Autodesk Fusion 360 part; units mm, degrees
note: some values were not read from the file. Chosen so that the rebuilt part matches the saved one: which bodies a step acts on.
(part 3 of 3)
  arc A214 (-6.6815, -293.4215) -> (-18.1828, -272.523) centre (-11.8765, -282.6665) cw
  arc A215 (-11.8752, -478.4075) -> (-10.2989, -476.8852) centre (3.5069, -492.7565) cw
  arc A216 (-159.2076, -214.1306) -> (-165.4906, -200.711) centre (-150.5091, -201.8774) cw
  arc A217 (-116.8581, -195.2756) -> (-109.0263, -217.8093) centre (-113.5449, -206.7519) cw
  arc A218 (-10.2989, -476.8852) -> (14.3752, -490.0489) centre (-0.5458, -488.3104) cw
  arc A219 (-16.473, -529.8025) -> (-27.9743, -508.904) centre (-21.668, -519.0474) cw
  arc A220 (47.4338, -419.9097) -> (41.1509, -406.49) centre (56.1324, -407.6565) cw
  arc A221 (-141.5323, -182.1119) -> (-116.8581, -195.2756) centre (-131.7791, -193.5371) cw
  arc A222 (-90.0824, -111.7167) -> (-76.5895, -97.9367) centre (-75.1054, -112.8859) cw
  arc A223 (-83.7995, -125.1364) -> (-90.0824, -111.7167) centre (-75.1009, -112.8832) cw
  line L0 (-266.5509, -596.9) -> (-266.5509, 0)
  arc A224 (266.8491, -596.9) -> (-266.5509, -596.9) centre (0.1491, -596.9) cw
  line L1 (266.8491, 0) -> (266.8491, -596.9)
  line L2 (241.4491, 0) -> (266.8491, 0)
  line L3 (-241.1509, 0) -> (-241.1509, -411.8539)
  arc A225 (-241.1509, -596.9) -> (241.4491, -596.9) centre (0.1491, -596.9) ccw
  line L4 (-241.1509, -439.1647) -> (-241.1509, -596.9)
  line L5 (241.4491, -596.9) -> (241.4491, 0)
  line L6 (-215.7509, -25.4) -> (-215.7509, -420.1147)
  arc A226 (-215.7509, -596.9) -> (216.0491, -596.9) centre (0.1491, -596.9) ccw
  line L7 (216.0491, -596.9) -> (216.0491, -25.4)
  line L8 (-215.7509, -439.1647) -> (-215.7509, -596.9)
  line L9 (-190.3509, -50.8) -> (-190.3509, -420.1147)
  line L10 (190.6491, -596.9) -> (190.6491, -50.8)
  line L11 (-190.3509, -439.1647) -> (-190.3509, -596.9)
  arc A227 (-190.3509, -596.9) -> (190.6491, -596.9) centre (0.1491, -596.9) ccw
  line L12 (216.0491, -25.4) -> (-215.7509, -25.4)
  line L13 (190.6491, -50.8) -> (-190.3509, -50.8)
  circle A228 centre (-203.0509, -429.6397) radius 6.35
  line L14 (-260.2009, -411.8539) -> (-241.1509, -411.8539)
  line L15 (-241.1509, -411.8539) -> (-241.1509, -428.0522)
  line L16 (-241.1509, -428.0522) -> (-260.2009, -428.0522)
  line L17 (-260.2009, -428.0522) -> (-260.2009, -411.8539)
  arc A229 (-152.1305, -436.5446) -> (-151.004, -435.1368) centre (-151.705, -435.7305) ccw
  line L18 (-261.7725, -439.1647) -> (-186.7302, -439.1647)
  arc A230 (-184.4429, -438.341) -> (-152.1305, -436.5446) centre (-167.2009, -456.9736) cw
  line L19 (-260.2009, -420.1147) -> (-261.7725, -420.1147)
  line L20 (-181.8374, -420.1147) -> (-241.1509, -420.1147)
  arc A231 (-151.004, -435.1368) -> (-181.8374, -420.1147) centre (-180.7971, -457.1339) ccw
  arc A232 (-261.7725, -420.1147) -> (-261.7725, -439.1647) centre (-236.358, -429.6397) ccw
  arc A233 (-186.7302, -439.1647) -> (-184.4429, -438.341) centre (-186.7379, -435.5556) ccw
  line L21 (222.3991, -25.4) -> (235.0991, -25.4)
  line L22 (235.0991, -25.4) -> (235.0991, -101.6)
  line L23 (235.0991, -101.6) -> (222.3991, -101.6)
  line L24 (222.3991, -101.6) -> (222.3991, -25.4)
  line L25 (222.3991, -63.5) -> (235.0991, -63.5)
  line L26 (216.0491, -25.4) -> (216.0491, -63.5)
  line L27 (216.0491, -63.5) -> (222.3991, -63.5)
  line L28 (222.3991, -63.5) -> (222.3991, -25.4)
  line L29 (222.3991, -25.4) -> (216.0491, -25.4)
  line L30 (235.0991, -101.6) -> (241.4491, -101.6)
  line L31 (235.0991, -63.5) -> (235.0991, -101.6)
  line L32 (241.4491, -63.5) -> (235.0991, -63.5)
  line L33 (241.4491, -101.6) -> (241.4491, -63.5)
  line L34 (222.3991, -518.7254) -> (235.0991, -518.7254)
  line L35 (235.0991, -594.9254) -> (222.3991, -594.9254)
  line L36 (222.3991, -594.9254) -> (222.3991, -518.7254)
  line L37 (235.0991, -518.7254) -> (235.0991, -594.9254)
  line L38 (222.3991, -556.8254) -> (235.0991, -556.8254)
  line L39 (216.0491, -518.7254) -> (216.0491, -556.8254)
  line L40 (222.3991, -556.8254) -> (222.3991, -518.7254)
  line L41 (222.3991, -518.7254) -> (216.0491, -518.7254)
  line L42 (216.0491, -556.8254) -> (222.3991, -556.8254)
  line L43 (241.4491, -556.8254) -> (235.0991, -556.8254)
  line L44 (235.0991, -556.8254) -> (235.0991, -594.9254)
  line L45 (235.0991, -594.9254) -> (241.4491, -594.9254)
  line L46 (241.4491, -594.9254) -> (241.4491, -556.8254)
  line L47 (6.4991, -50.8) -> (6.4991, -237.1607)
  line L48 (6.4991, -242.0445) -> (6.4991, -277.5095)
  line L49 (6.4991, -282.0442) -> (6.4991, -295.7652)
  line L50 (6.4991, -300.6585) -> (6.4991, -475.0428)
  line L51 (6.4991, -480.8522) -> (6.4991, -496.4423)
  line L52 (6.4991, -512.5757) -> (6.4991, -522.9778)
  line L53 (6.4991, -528.6458) -> (6.4991, -787.2941)
  line L54 (-6.2009, -50.8) -> (-6.2009, -244.5718)
  line L55 (-6.2009, -249.5407) -> (-6.2009, -272.1568)
  line L56 (-6.2009, -278.266) -> (-6.2009, -287.0667)
  line L57 (-6.2009, -294.4545) -> (-6.2009, -474.3935)
  line L58 (-6.2009, -479.7502) -> (-6.2009, -514.0409)
  line L59 (-6.2009, -518.147) -> (-6.2009, -532.4242)
  line L60 (-6.2009, -537.2039) -> (-6.2009, -787.2941)
  line L61 (-59.1175, -50.8) -> (-59.1175, -89.7741)
  line L62 (-59.1175, -94.6578) -> (-59.1175, -130.1228)
  line L63 (-59.1175, -134.6575) -> (-59.1175, -148.3785)
  line L64 (-59.1175, -153.2719) -> (-59.1175, -327.6562)
  line L65 (-59.1175, -333.4655) -> (-59.1175, -349.0556)
  line L66 (-59.1175, -365.1891) -> (-59.1175, -375.5911)
  line L67 (-59.1175, -381.2592) -> (-59.1175, -777.9462)
  line L68 (-71.8175, -50.8) -> (-71.8175, -97.1851)
  line L69 (-71.8175, -102.1541) -> (-71.8175, -124.5061)
  line L70 (-71.8175, -130.8793) -> (-71.8175, -139.68)
  line L71 (-71.8175, -147.0678) -> (-71.8175, -327.0069)
  line L72 (-71.8175, -332.3636) -> (-71.8175, -366.6542)
  line L73 (-71.8175, -370.7604) -> (-71.8175, -385.0376)
  line L74 (-71.8175, -389.8173) -> (-71.8175, -773.2832)
  line L75 (72.1158, -50.8) -> (72.1158, -384.5474)
  line L76 (72.1158, -389.4311) -> (72.1158, -424.8962)
  line L77 (72.1158, -429.4308) -> (72.1158, -443.1518)
  line L78 (72.1158, -448.0452) -> (72.1158, -622.4295)
  line L79 (72.1158, -628.2388) -> (72.1158, -643.8289)
  line L80 (72.1158, -659.9624) -> (72.1158, -670.3644)
  line L81 (72.1158, -676.0325) -> (72.1158, -773.2832)
  line L82 (59.4158, -50.8) -> (59.4158, -391.9584)
  line L83 (59.4158, -396.9274) -> (59.4158, -419.5435)
  line L84 (59.4158, -425.6526) -> (59.4158, -434.4533)
  line L85 (59.4158, -441.8411) -> (59.4158, -621.7802)
  line L86 (59.4158, -627.1369) -> (59.4158, -661.4275)
  line L87 (59.4158, -665.5337) -> (59.4158, -679.8109)
  line L88 (59.4158, -684.5906) -> (59.4158, -777.9462)
  line L89 (137.7325, -50.8) -> (137.7325, -531.934)
  line L90 (137.7325, -536.8178) -> (137.7325, -572.2828)
  line L91 (137.7325, -576.8175) -> (137.7325, -590.5385)
  line L92 (137.7325, -595.4318) -> (137.7325, -728.6614)
  line L93 (125.0325, -50.8) -> (125.0325, -539.3451)
  line L94 (125.0325, -544.314) -> (125.0325, -566.6661)
  line L95 (125.0325, -573.0393) -> (125.0325, -581.84)
  line L96 (125.0325, -589.2278) -> (125.0325, -740.7555)
  line L97 (-124.7342, -50.8) -> (-124.7342, -180.2695)
  line L98 (-124.7342, -186.0789) -> (-124.7342, -201.669)
  line L99 (-124.7342, -217.8024) -> (-124.7342, -228.2045)
  line L100 (-124.7342, -233.8725) -> (-124.7342, -740.7555)
  line L101 (-137.4342, -50.8) -> (-137.4342, -179.6202)
  line L102 (-137.4342, -184.9769) -> (-137.4342, -219.2676)
  line L103 (-137.4342, -223.3737) -> (-137.4342, -237.6509)
  line L104 (-137.4342, -242.4306) -> (-137.4342, -728.6614)
  line L105 (284.6029, 0) -> (-289.1743, 0)
extrude "Extrude5" add sketch "DJ - Baxley - Dog Door (1) (curves -6.35 mm off its plane)" against normal blind 6.35 separate body contours A8 A16 A62 A142 A214 | A8 A54 A142 L55 | A8 A32 A43 A48 A50 A54 A62 A63 A76 A99 A102 A112 A113 A115 A176 A177 A188 A191 A193 A196 A211 L55 | A8 A16 A32 A146 | A8 A16 A32 A62 | A10 A35 A45 A58 A65 A68 A69 A74 A77 A87 A88 A96 A106 A107 A121 A152 A155 A199 A200 A212 A215 A218 | A16 A32 A43 A62 A207 | A17 A35 A45 A121 A210 | A9 A39 A47 A109 A111 A118 A119 A120 A123 A126 A136 A137 A139 A140 A143 A169 A185 A189 A192 A194 A222 A223 | A12 A34 A41 A64 A66 A67 A70 A80 A81 A90 A93 A95 A103 A117 A144 A150 A203 A208 A209 A213 A220 L83 | A10 A17 A35 A153 | A10 A17 A87 A121 A219 | A14 A38 A46 A110 A114 A116 A122 A124 A125 A127 A130 A131 A132 A133 A135 A174 A201 A205 A206 A216 A217 A221 | A22 A39 A47 A109 A171 | A10 A17 A35 A121 | A13 A36 A44 A51 A59 A60 A73 A75 A84 A86 A97 A98 A101 A105 A128 A147 A148 A151 A158 A161 A164 A170 | A11 A19 A33 A162 | A20 A34 A41 A70 A154 | A21 A38 A46 A124 A198 | A9 A22 A39 A195 | A23 A37 A40 A55 A183 | A19 A33 A42 A53 A163 | A11 A19 A49 A53 A168 | A12 A20 A70 A91 A202 | A9 A22 A109 A123 A197 | A15 A23 A37 A182 | A13 A18 A36 A160 | A11 A33 A42 A49 A52 A53 A71 A78 A82 A83 A94 A100 A104 A138 A141 A145 A149 A156 A157 A159 A165 A167 | A18 A36 A44 A73 A172 | A12 A20 A34 A204 | A12 A81 A91 L83 | A9 A22 A39 A109 | A15 A37 A40 A55 A56 A57 A61 A72 A79 A85 A89 A92 A108 A129 A134 A173 A175 A179 A180 A181 A187 A190 | A15 A23 A55 A61 A184 | A13 A18 A73 A128 A166 | A11 A19 A33 A53 | A14 A21 A38 A186 | A15 A23 A37 A55 | A12 A20 A34 A70 | A14 A21 A38 A124 | A14 A21 A124 A135 A178 | A13 A18 A36 A73 makes body 4 at (76.4475, -6.35, 427.4285) makes body 5 at (1.0394, -6.35, 516.4228) makes body 6 at (10.8309, -6.35, 280.0418) makes body 7 at (142.0642, -6.35, 574.8151) makes body 8 at (-64.5773, -6.35, 369.0361) makes body 9 at (-130.1939, -6.35, 221.6495) makes body 10 at (66.6561, -6.35, 663.8094) makes body 11 at (-54.7858, -6.35, 132.6552)
sketch "Sketch5" plane through (0, 0, 0) normal (0, 1, 0) x (1, 0, 0)
  arc A0 through (-152.1305, -436.5446, -12.7) (-150.9878, -436.3044, -12.7) (-151.004, -435.1368, -12.7)
  line L0 (-190.3509, -439.1647, -12.7) -> (-190.3509, -596.9, -12.7)
  line L1 (-241.1509, -439.1647, -12.7) -> (-241.1509, -596.9, -12.7)
  line L2 (-190.3509, -50.8, -12.7) -> (-190.3509, -420.1147, -12.7)
  line L3 (-241.1509, 0, -12.7) -> (-241.1509, -411.8539, -12.7)
  line L4 (-215.7509, -25.4, -12.7) -> (-215.7509, -420.1147, -12.7)
  circle A1 through (-209.4009, -429.6397, -12.7) (-199.8759, -424.1405, -12.7) (-199.8759, -435.139, -12.7)
  line L5 (-215.7509, -420.1147, -12.7) -> (-215.7509, -439.1647, -12.7)
  line L6 (-253.8509, -428.0522, -12.7) -> (-253.8509, -411.8539, -12.7)
  line L7 (-181.8374, -420.1147, -12.7) -> (-241.1509, -420.1147, -12.7)
  line L8 (-241.1509, -428.0522, -12.7) -> (-253.8509, -428.0522, -12.7)
  line L9 (-255.4225, -439.1647, -12.7) -> (-186.7302, -439.1647, -12.7)
  arc A2 through (-151.004, -435.1368, -12.7) (-164.5769, -423.8412, -12.7) (-181.8374, -420.1147, -12.7)
  arc A3 through (-152.1305, -436.5446, -12.7) (-150.9878, -436.3044, -12.7) (-151.004, -435.1368, -12.7)
  line L10 (-253.8509, -411.8539, -12.7) -> (-241.1509, -411.8539, -12.7)
  line L11 (-241.1509, -428.0522, -12.7) -> (-241.1509, -439.1647, -12.7)
  arc A4 through (-186.7302, -439.1647, -12.7) (-185.5151, -438.9513, -12.7) (-184.4429, -438.341, -12.7)
  arc A5 through (-255.4225, -420.1147, -12.7) (-257.1487, -429.6397, -12.7) (-255.4225, -439.1647, -12.7)
  arc A6 through (-184.4429, -438.341, -12.7) (-168.61, -431.6265, -12.7) (-152.1305, -436.5446, -12.7)
  line L12 (-241.1509, -411.8539, -12.7) -> (-241.1509, -428.0522, -12.7)
  line L13 (-190.3509, -439.1647, -12.7) -> (-190.3509, -420.1147, -12.7)
  line L14 (-253.8509, -420.1147, -12.7) -> (-255.4225, -420.1147, -12.7)
  line L15 (-215.7509, -439.1647, -12.7) -> (-215.7509, -596.9, -12.7)
  line L16 (-253.8509, -420.1147, -12.7) -> (-241.1509, -420.1147, -12.7)
sketch "Sketch6" plane through (0, 0, 0) normal (0, 1, 0) x (1, 0, 0)
  line L0 (222.3991, -63.5) -> (222.3991, -25.4)
  line L1 (222.3991, -101.6) -> (222.3991, -25.4)
  line L2 (235.0991, -25.4) -> (235.0991, -101.6)
  line L3 (235.0991, -101.6) -> (222.3991, -101.6)
  line L4 (222.3991, -25.4) -> (235.0991, -25.4)
  line L5 (216.0491, -63.5) -> (222.3991, -63.5)
  line L6 (216.0491, -25.4) -> (216.0491, -63.5)
  line L7 (222.3991, -25.4) -> (216.0491, -25.4)
  line L8 (241.4491, -63.5) -> (235.0991, -63.5)
  line L9 (235.0991, -101.6) -> (241.4491, -101.6)
  line L10 (235.0991, -594.9254) -> (222.3991, -594.9254)
  line L11 (235.0991, -518.7254) -> (235.0991, -594.9254)
  line L12 (222.3991, -594.9254) -> (222.3991, -518.7254)
  line L13 (222.3991, -518.7254) -> (235.0991, -518.7254)
  line L14 (222.3991, -556.8254) -> (235.0991, -556.8254)
  line L15 (241.4491, -556.8254) -> (235.0991, -556.8254)
  line L16 (216.0491, -556.8254) -> (222.3991, -556.8254)
  line L17 (222.3991, -518.7254) -> (216.0491, -518.7254)
  line L18 (235.0991, -594.9254) -> (241.4491, -594.9254)
  line L19 (241.4491, -594.9254) -> (241.4491, -556.8254)
  line L20 (216.0491, -556.8254) -> (216.0491, -518.7254)
  line L21 (241.4491, -101.6) -> (241.4491, -63.5)
  line L22 (228.7491, -101.6) -> (228.7491, -25.4)
  line L23 (228.7491, -594.9254) -> (228.7491, -518.7254)
  point P0 (222.3991, -556.8254)
  constraint coincident L18.end L19.start
  constraint coincident L15.start L19.end
  constraint coincident L16.start L20.start
  constraint coincident L17.end L20.end
  constraint coincident L9.end L21.start
  constraint coincident L8.start L21.end
  constraint midpoint L3 L22.start
  constraint midpoint L4 L22.end
  constraint midpoint L10 L23.start
  constraint perpendicular L13 L23
revolve "Revolve1" add sketch "Sketch6" angle 360 about axis through (228.7491, 0, 101.6) along (0, 0, -1) separate body contours L2 L3 L4 L22 | L10 L11 L14 L23 | L11 L13 L14 L23 makes body 12 at (230.7715, -6.0193, 544.1254) makes body 13 at (230.7715, -6.0193, 50.8)
extrude "Extrude6" add sketch "Sketch6" along normal mid plane 3.048 separate body contours L0 L1 L5 L6 L7 | L2 L8 L9 L21 | L11 L15 L18 L19 | L12 L16 L17 L20 makes body 14 at (237.2158, 1.524, 569.5254) makes body 15 at (220.2825, 1.524, 50.8) makes body 16 at (218.1658, 1.524, 544.1254) makes body 17 at (237.2158, 1.524, 76.2)
combine "Combine1" operation add target body 17 tool bodies 15 13
combine "Combine2" operation add target body 14 tool bodies 12 16
sketch "Sketch5 (curves -12.7 mm off its plane)" plane through (0, -12.7, 0) normal (0, 1, 0) x (1, 0, 0)
  arc A0 (-152.1305, -436.5446) -> (-151.004, -435.1368) centre (-151.705, -435.7305) ccw
  line L0 (-190.3509, -439.1647) -> (-190.3509, -596.9)
  line L1 (-241.1509, -439.1647) -> (-241.1509, -596.9)
  line L2 (-190.3509, -50.8) -> (-190.3509, -420.1147)
  line L3 (-241.1509, 0) -> (-241.1509, -411.8539)
  line L4 (-215.7509, -25.4) -> (-215.7509, -420.1147)
  circle A1 centre (-203.0509, -429.6397) radius 6.35
  line L5 (-215.7509, -420.1147) -> (-215.7509, -439.1647)
  line L6 (-253.8509, -428.0522) -> (-253.8509, -411.8539)
  line L7 (-181.8374, -420.1147) -> (-241.1509, -420.1147)
  line L8 (-241.1509, -428.0522) -> (-253.8509, -428.0522)
  line L9 (-255.4225, -439.1647) -> (-186.7302, -439.1647)
  arc A2 (-151.004, -435.1368) -> (-181.8374, -420.1147) centre (-180.7971, -457.1339) ccw
  arc A3 (-152.1305, -436.5446) -> (-151.004, -435.1368) centre (-151.705, -435.7305) ccw
  line L10 (-253.8509, -411.8539) -> (-241.1509, -411.8539)
  line L11 (-241.1509, -428.0522) -> (-241.1509, -439.1647)
  arc A4 (-186.7302, -439.1647) -> (-184.4429, -438.341) centre (-186.7379, -435.5556) ccw
  arc A5 (-255.4225, -420.1147) -> (-255.4225, -439.1647) centre (-230.008, -429.6397) ccw
  arc A6 (-184.4429, -438.341) -> (-152.1305, -436.5446) centre (-167.2009, -456.9736) cw
  line L12 (-241.1509, -411.8539) -> (-241.1509, -428.0522)
  line L13 (-190.3509, -439.1647) -> (-190.3509, -420.1147)
  line L14 (-253.8509, -420.1147) -> (-255.4225, -420.1147)
  line L15 (-215.7509, -439.1647) -> (-215.7509, -596.9)
  line L16 (-253.8509, -420.1147) -> (-241.1509, -420.1147)
extrude "Extrude7" add sketch "Sketch5 (curves -12.7 mm off its plane)" along normal blind 3.175 from surface at -6.35 separate body contours A0 L7 L9 A2 A3 A4 A6 L13 | L5 L7 L9 L13 | L5 L7 L9 L11 L12 | L6 L8 L12 L16 | L6 L8 L9 L11 A5 L14 makes body 18
extrude "Extrude8" add sketch "Sketch5 (curves -12.7 mm off its plane)" against normal blind 9.525 separate body contours A1 makes body 19
extrude "Extrude9" add sketch "Sketch5 (curves -12.7 mm off its plane)" against normal blind 9.525 separate body contours L6 L10 L12 L16 | L6 L8 L12 L16 makes body 20
extrude "Extrude10" cut sketch "Sketch5 (curves -12.7 mm off its plane)" against normal blind 6.985 contours L6 L8 L12 L16 bodies 20
fillet "Fillet1" radius 3.175 1 edges at (-197.1306, -22.225, 431.936) on bodies 19
